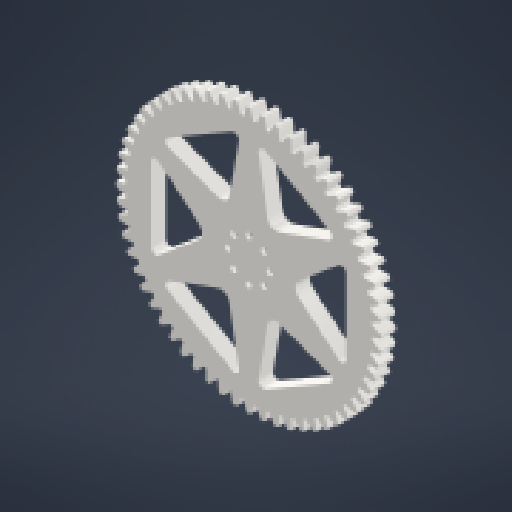
# Autodesk Inventor part: Spur Gear2
Saved by Autodesk Inventor 2023 (Build 270158000, 158)
## iProperties
CustomPartVersion: 1
Created: 2022-11-12
Part Number: Spur Gear2
Material: Steel
Document SubType Name: Modeling
Designer: izack
Categories: <?xml version="1.0" encoding="UTF-16"?> <MemberInstance><Categories><FamilyTemplate><FamilyTemplateParameter ValueType="xs:double" Id="1" ObjectReferenceKey="da_z" ObjectType="kUserParameterObject"/><FamilyTemplateParameter ValueType="xs:double" Id="2" ObjectReferenceKey="da_b" ObjectType="kUserParameterObject"/><FamilyTemplateParameter ValueType="xs:double" Id="3" ObjectReferenceKey="da_beta" ObjectType="kUserParameterObject"/><FamilyTemplateParameter ValueType="xs:double" Id="4" ObjectReferenceKey="da_da" ObjectType="kUserParameterObject"/><FamilyTemplateParameter ValueType="xs:double" Id="5" ObjectReferenceKey="da_aw" ObjectType="kUserParameterObject"/><FamilyTemplateParameter ValueType="xs:string" Id="6" ObjectReferenceKey="EAIAABAAAACIAQAAAAAAAIAAAAAAAAAA" ObjectType="83910656" SubObjectId="SurfaceGeometry"/></FamilyTemplate><ParamToTemplateMap><ParamToTemplate CategoryParameter="//CategoryParameter[@InternalName='046C89C9-8512-4d59-83FE-43B91F4F132A']" TemplateParameter="1"/><ParamToTemplate CategoryParameter="//CategoryParameter[@InternalName='2552DF32-E462-4b46-AEBF-C6C7768E72AC']" TemplateParameter="2"/><ParamToTemplate CategoryParameter="//CategoryParameter[@InternalName='C9EE641D-15FC-4fae-A226-E94C4372FDD7']" TemplateParameter="3"/><ParamToTemplate><ParamToTemplate CategoryParameter="//CategoryParameter[@InternalName='00B6519A-459B-49c7-AD84-2E56D39A5744']" ConstantValue="0.000000"/></ParamToTemplate><ParamToTemplate><ParamToTemplate CategoryParameter="//CategoryParameter[@InternalName='04B31F0E-C7A6-4894-AA32-9629BEFACF47']" ConstantValue="1.000000"/></ParamToTemplate><ParamToTemplate><ParamToTemplate CategoryParameter="//CategoryParameter[@InternalName='43CBEC2E-7847-49e7-A936-2F7889FCB2D9']" ConstantValue="0.250000"/></ParamToTemplate><ParamToTemplate><ParamToTemplate CategoryParameter="//CategoryParameter[@InternalName='B1EFC894-105D-4ebd-86BF-FA20ED196853']" ConstantValue="0.350000"/></ParamToTemplate><ParamToTemplate><ParamToTemplate CategoryParameter="//CategoryParameter[@InternalName='51175063-3D10-4879-93E8-6246FE8B403D']" ConstantValue="2060000000.000000"/></ParamToTemplate><ParamToTemplate><ParamToTemplate CategoryParameter="//CategoryParameter[@InternalName='A3A52E27-4454-46a9-B0BD-C932399B70AF']" ConstantValue="0.300000"/></ParamToTemplate><ParamToTemplate><ParamToTemplate CategoryParameter="//CategoryParameter[@InternalName='91B76062-C214-41d9-B1B9-14D2AB99603D']" ConstantValue="0.230000"/></ParamToTemplate><ParamToTemplate><ParamToTemplate CategoryParameter="//CategoryParameter[@InternalName='374E806E-8B8A-4dda-A9AA-1039D6500AD2']" ConstantValue="4.347826"/></ParamToTemplate><ParamToTemplate><ParamToTemplate CategoryParameter="//CategoryParameter[@InternalName='2D373A89-B862-43d6-8D0B-0CBF12AB9F6C']" ConstantValue="0.349066"/></ParamToTemplate><ParamToTemplate CategoryParameter="//CategoryParameter[@InternalName='37777632-D6A2-4fac-9D53-DB8ACD95C989']" TemplateParameter="4"/><ParamToTemplate CategoryParameter="//CategoryParameter[@InternalName='FD1017F1-B727-4f7e-9707-0F86F1FF9423']" TemplateParameter="5"/><ParamToTemplate><ParamToTemplate CategoryParameter="//CategoryParameter[@InternalName='9E1B4470-B2D3-4ff1-B813-535BB4CDF51A']" ConstantValue="3520000.000000"/></ParamToTemplate><ParamToTemplate><ParamToTemplate CategoryParameter="//CategoryParameter[@InternalName='F8452263-BFF6-458c-9FB1-07C4B99E95CD']" ConstantValue="11400000.000000"/></ParamToTemplate><ParamToTemplate><ParamToTemplate CategoryParameter="//CategoryParameter[@InternalName='3E3BB259-FD49-497f-8171-6EBC954A3479']" ConstantValue="2.000000"/></ParamToTemplate><ParamToTemplate CategoryParameter="//CategoryParameter[@InternalName='27C3BAF2-7550-4e4b-AE2C-0DB134B7D9B7']" TemplateParameter="6"/></ParamToTemplateMap><Category DisplayName="Gear" InternalName="DC85795E-93AB-48d5-8EEE-5A27447B64BD" Mnemonic="Gear"><CategoryParameter DisplayName="z" InternalName="046C89C9-8512-4d59-83FE-43B91F4F132A" Mnemonic="z"/><CategoryParameter DisplayName="b" InternalName="2552DF32-E462-4b46-AEBF-C6C7768E72AC" Mnemonic="b"/><CategoryParameter DisplayName="||b|" InternalName="C9EE641D-15FC-4fae-A226-E94C4372FDD7" Mnemonic="beta"/><CategoryParameter DisplayName="x" InternalName="00B6519A-459B-49c7-AD84-2E56D39A5744" Mnemonic="x"/><CategoryParameter DisplayName="a*" InternalName="04B31F0E-C7A6-4894-AA32-9629BEFACF47" Mnemonic="a"/><CategoryParameter DisplayName="c*" InternalName="43CBEC2E-7847-49e7-A936-2F7889FCB2D9" Mnemonic="c"/><CategoryParameter DisplayName="r|.f|*" InternalName="B1EFC894-105D-4ebd-86BF-FA20ED196853" Mnemonic="rf"/><CategoryParameter DisplayName="E" InternalName="51175063-3D10-4879-93E8-6246FE8B403D" Mnemonic="E"/><CategoryParameter DisplayName="||m|" InternalName="A3A52E27-4454-46a9-B0BD-C932399B70AF" Mnemonic="mi"/><Category DisplayName="SpurGear" InternalName="26C5A22E-A91E-4dfd-A3B3-23CCAFAE1764" Mnemonic="SpurGear"><CategoryParameter DisplayName="m" InternalName="91B76062-C214-41d9-B1B9-14D2AB99603D" Mnemonic="m"/><CategoryParameter DisplayName="P" InternalName="374E806E-8B8A-4dda-A9AA-1039D6500AD2" Mnemonic="PP"/><CategoryParameter DisplayName="||a|" InternalName="2D373A89-B862-43d6-8D0B-0CBF12AB9F6C" Mnemonic="alpha"/><CategoryParameter DisplayName="d|.a|" InternalName="37777632-D6A2-4fac-9D53-DB8ACD95C989" Mnemonic="da"/><CategoryParameter DisplayName="a|.w|" InternalName="FD1017F1-B727-4f7e-9707-0F86F1FF9423" Mnemonic="aw"/><CategoryParameter DisplayName="||s||.Flim|" InternalName="9E1B4470-B2D3-4ff1-B813-535BB4CDF51A" Mnemonic="sFlim"/><CategoryParameter DisplayName="||s||.Hlim|" InternalName="F8452263-BFF6-458c-9FB1-07C4B99E95CD" Mnemonic="sHlim"/><CategoryParameter DisplayName="type" InternalName="3E3BB259-FD49-497f-8171-6EBC954A3479" Mnemonic="type"/><CategoryParameter DisplayName="PitchDiameter" InternalName="27C3BAF2-7550-4e4b-AE2C-0DB134B7D9B7" Mnemonic="IDS_PITCHDIAM"/></Category></Category></Categories></MemberInstance>
Density: 1 g/cm^3
Appearance: Steel
Author: izack
Autodesk Inventor part; units mm, degrees
ref_plane "YZ Plane" through (0, 0, 0) normal (1, 0, 0) x (0, 1, 0)
ref_plane "XZ Plane" through (0, 0, 0) normal (0, 1, 0) x (-1, 0, 0)
ref_plane "XY Plane" through (0, 0, 0) normal (0, 0, 1) x (1, 0, 0)
sketch "Sketch1" plane through (0, 0, 0) normal (0, 0, 1) x (1, 0, 0)
  circle A0 centre (0, 0) radius 71.3
  dimension "d0" = 142.6
  constraints: 1 centre point
  measures "d0" diameter of A0
extrude "Extrusion1" add sketch "Sketch1" along normal blind 8
ref_plane "Work Plane2" through (0, 0, 4) normal (0, 0, 1) x (1, 0, 0)
sketch "Sketch2" plane through (0, 0, 0) normal (0, 0, -1) x (-1, 0, 0)
  circle A0 centre (0, 0) radius 71.3 projected
  circle A1 centre (0, 0) radius 69
  dimension "d3" = 138
  constraints: 1 centre point, 1 coincident
  measures "d3" diameter of A1
surface extrude "Pitch Diameter" sketch "Sketch2" against normal through all shown no curves A1
ref_plane "Work Plane8" through (0, 0, 0) normal (0.9986295, 0.052336, 0) x (0, 0, 1)
ref_plane "Work Plane9" through (0, 0, 0) normal (1, 0, 0) x (0, 1, 0)
spur gear teeth "Spur Gear" teeth 60 pitch diameter 138 tip diameter 142.6 root diameter 132.25 face width 8 start plane through (0, 0, 0) normal (0, 0, -1) x (-1, 0, 0)
sketch "Sketch3" plane through (0, 0, 0) normal (0, 0, -1) x (-1, 0, 0)
  circle A0 centre (0, 0) radius 16.5
  dimension "d49" = 33
  constraints: 1 centre point, 1 coincident
  measures "d49" diameter of A0
extrude "Extrusion2" cut sketch "Sketch3" against normal blind 6
sketch "Sketch4" plane through (0, 0, 8) normal (0, 0, 1) x (1, 0, 0)
  circle A0 centre (0, 0) radius 11.315
  circle A1 centre (11.315, 0) radius 1.7
  circle A2 centre (8.0009, 8.0009) radius 1.7
  circle A3 centre (0, 11.315) radius 1.7
  circle A4 centre (-8.0009, 8.0009) radius 1.7
  circle A5 centre (-11.315, 0) radius 1.7
  circle A6 centre (-8.0009, -8.0009) radius 1.7
  circle A7 centre (0, -11.315) radius 1.7
  circle A8 centre (8.0009, -8.0009) radius 1.7
  dimension "d52" = 22.63
  dimension "d53" = 3.4
  dimension "d56" = 360
  constraints: 8 centre point, 1 coincident, 1 horizontal alignment, 19 other
  measures "d53" diameter of A1
extrude "Extrusion3" cut sketch "Sketch4" against normal blind 6 contours A0 A1 | A0 A1 | A2 A0 | A0 A2 | A8 A0 | A0 A8 | A3 A0 | A0 A3 | A7 A0 | A0 A7 | A4 A0 | A0 A4 | A6 A0 | A0 A6 | A5 A0 | A0 A5
sketch "Sketch5" plane through (0, 0, 8) normal (0, 0, 1) x (1, 0, 0)
  circle A0 centre (0, 0) radius 22.5
  circle A1 centre (0, 0) radius 55
  arc A2 (52.5, 20) -> (48.3954, 21.9171) centre (50, 20) ccw
  arc A3 (48.3954, -21.9171) -> (52.5, -20) centre (50, -20) ccw
  arc A4 (26.7908, 3.8342) -> (26.7908, -3.8342) centre (30, 0) ccw
  line L0 (50, 20) -> (50, -20) construction
  line L1 (0, 0) -> (73.7278, 0) construction
  line L2 (48.3954, 21.9171) -> (26.7908, 3.8342)
  line L3 (52.5, 20) -> (52.5, -20)
  line L4 (26.7908, -3.8342) -> (48.3954, -21.9171)
  arc A5 (43.1785, 30.9531) -> (43.5705, 35.4663) centre (42.3205, 33.3013) ccw
  arc A6 (10.0749, 25.1186) -> (16.7159, 21.2844) centre (15, 25.9808) ccw
  line L5 (7.6795, 53.3013) -> (42.3205, 33.3013) construction
  line L6 (8.9295, 55.4663) -> (43.5705, 35.4663)
  line L7 (5.2169, 52.8702) -> (10.0749, 25.1186)
  arc A7 (8.9295, 55.4663) -> (5.2169, 52.8702) centre (7.6795, 53.3013) ccw
  line L8 (16.7159, 21.2844) -> (43.1785, 30.9531)
  arc A8 (-5.2169, 52.8702) -> (-8.9295, 55.4663) centre (-7.6795, 53.3013) ccw
  arc A9 (-16.7159, 21.2844) -> (-10.0749, 25.1186) centre (-15, 25.9808) ccw
  line L9 (-42.3205, 33.3013) -> (-7.6795, 53.3013) construction
  line L10 (-43.5705, 35.4663) -> (-8.9295, 55.4663)
  line L11 (-43.1785, 30.9531) -> (-16.7159, 21.2844)
  arc A10 (-43.5705, 35.4663) -> (-43.1785, 30.9531) centre (-42.3205, 33.3013) ccw
  line L12 (-10.0749, 25.1186) -> (-5.2169, 52.8702)
  arc A11 (-48.3954, 21.9171) -> (-52.5, 20) centre (-50, 20) ccw
  arc A12 (-26.7908, -3.8342) -> (-26.7908, 3.8342) centre (-30, 0) ccw
  line L13 (-50, -20) -> (-50, 20) construction
  line L14 (-52.5, -20) -> (-52.5, 20)
  line L15 (-48.3954, -21.9171) -> (-26.7908, -3.8342)
  arc A13 (-52.5, -20) -> (-48.3954, -21.9171) centre (-50, -20) ccw
  line L16 (-26.7908, 3.8342) -> (-48.3954, 21.9171)
  arc A14 (-43.1785, -30.9531) -> (-43.5705, -35.4663) centre (-42.3205, -33.3013) ccw
  arc A15 (-10.0749, -25.1186) -> (-16.7159, -21.2844) centre (-15, -25.9808) ccw
  line L17 (-7.6795, -53.3013) -> (-42.3205, -33.3013) construction
  line L18 (-8.9295, -55.4663) -> (-43.5705, -35.4663)
  line L19 (-5.2169, -52.8702) -> (-10.0749, -25.1186)
  arc A16 (-8.9295, -55.4663) -> (-5.2169, -52.8702) centre (-7.6795, -53.3013) ccw
  line L20 (-16.7159, -21.2844) -> (-43.1785, -30.9531)
  arc A17 (5.2169, -52.8702) -> (8.9295, -55.4663) centre (7.6795, -53.3013) ccw
  arc A18 (16.7159, -21.2844) -> (10.0749, -25.1186) centre (15, -25.9808) ccw
  line L21 (42.3205, -33.3013) -> (7.6795, -53.3013) construction
  line L22 (43.5705, -35.4663) -> (8.9295, -55.4663)
  line L23 (43.1785, -30.9531) -> (16.7159, -21.2844)
  arc A19 (43.5705, -35.4663) -> (43.1785, -30.9531) centre (42.3205, -33.3013) ccw
  line L24 (10.0749, -25.1186) -> (5.2169, -52.8702)
  point P0 (50, 0)
  point P1 (25, 43.3013)
  point P2 (-25, 43.3013)
  point P3 (-50, 0)
  point P4 (-25, -43.3013)
  point P5 (25, -43.3013)
  dimension "d60" = 45
  dimension "d61" = 110
  dimension "d62" = 5
  dimension "d63" = 5
  dimension "d64" = 10
  dimension "d65" = 30
  dimension "d66" = 40
  dimension "d67" = 50
  dimension "d70" = 360
  constraints: 50 end point, 36 point on circle, 20 centre point, 14 coincident, 5 tangent, 2 point on line, 2 vertical, 1 horizontal, 1 midpoint, 115 other
  measures "d60" diameter of A0
  measures "d61" diameter of A1
  measures "d62" diameter of A2
  measures "d63" diameter of A3
  measures "d64" diameter of A4
  measures "d65" distance of point (0, 0) A4.centre
  measures "d66" distance of L0.start L0.end
  measures "d67" distance from line of point (0, 0) L0
extrude "Extrusion4" cut sketch "Sketch5" against normal through all contours L3 A1 A3 L4 A4 L2 A2 | A1 A2 L3 | L3 A3 A1 | A5 L8 A6 L7 A7 A1 L6 | A1 L6 A5 | A19 L22 A1 | A1 L22 A17 L24 A18 L23 A19 | A1 A7 L6 | L22 A17 A1 | A8 L12 A9 L11 A10 A1 L10 | A1 L10 A8 | A16 L18 A1 | A1 L18 A14 L20 A15 L19 A16 | A1 A10 L10 | L18 A14 A1 | A11 L16 A12 L15 A13 A1 L14 | A1 L14 A11 | A13 L14 A1
equation "\"d0\" = da_da"
equation "\"d1\" = da_b"
equation "\"d3\" = da_d"
equation "\"d16\" = da_aw"
equation "\"d43\" = da_aw"
equation "\"d46\" = da_aw"
equation "\"da_da\" = 142.6"
equation "\"da_b\" = 8"
equation "\"da_d\" = 138"
equation "\"da_aw\" = 126.5"
body "Solid1"
body "Srf1"
